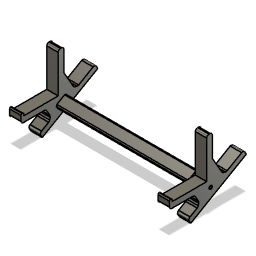
CHORDS Stand X2 (Autodesk Fusion 360 design; units mm, degrees)
Autodesk Fusion 360 part; units mm, degrees
sketch "Sketch1" plane through (0, 0, 0) normal (1, 0, 0) x (0, 0, -1)
  line L0 (0, 0) -> (-60, 0) construction
  line L1 (-60, 0) -> (-60, 138.5) construction
  line L2 (-60, 138.5) -> (0, 138.5) construction
  line L3 (0, 138.5) -> (0, 0) construction
  line L4 (0, 0) -> (-60, 0)
  line L5 (-60, 0) -> (-60.2, 0)
  line L6 (-60.2, 0) -> (-60.2, 5)
  line L7 (-60.2, 5) -> (-65.2, 5)
  line L8 (-65.2, 5) -> (-65.2, -10)
  line L9 (0, 0) -> (0, 70)
  line L10 (0, 70) -> (10, 70)
  line L11 (10, 70) -> (10, 30)
  line L12 (10, 30) -> (30, -4.641)
  line L13 (-65.2, -10) -> (-21.6, -10)
  line L14 (30, -4.641) -> (64.641, 15.359)
  line L15 (30, -4.641) -> (65.2811, -4.641) construction
  line L16 (30, -4.641) -> (-60.7782, -57.0519) construction
  line L17 (-21.6, -10) -> (-11.0205, -28.3242)
  line L18 (-11.0205, -28.3242) -> (-32.6711, -40.8242)
  line L19 (-32.6711, -40.8242) -> (-27.6711, -49.4845)
  line L20 (64.641, 15.359) -> (69.641, 6.6987)
  line L21 (69.641, 6.6987) -> (-27.6711, -49.4845)
  line L22 (0, 0) -> (14.5096, -25.1314) construction
  line L23 (14.5096, -25.1314) -> (9.5096, -16.4711) construction
  line L24 (9.5096, -16.4711) -> (18.1699, -11.4711)
  line L25 (18.1699, -11.4711) -> (13.1699, -2.8109)
  line L26 (13.1699, -2.8109) -> (4.5096, -7.8109)
  line L27 (-4.1506, -12.8109) -> (4.5096, -7.8109)
  line L28 (0.8494, -21.4711) -> (-4.1506, -12.8109)
  line L29 (9.5096, -16.4711) -> (0.8494, -21.4711)
  line L30 (-3.8774, -12.8841) -> (4.6096, -7.9841)
  line L31 (13.0967, -3.0841) -> (4.6096, -7.9841)
  line L32 (17.8967, -11.3979) -> (13.0967, -3.0841)
  line L33 (9.4096, -16.2979) -> (17.8967, -11.3979)
  line L34 (9.4096, -16.2979) -> (0.9226, -21.1979)
  line L35 (0.9226, -21.1979) -> (-3.8774, -12.8841)
  line L36 (4.5096, -7.8109) -> (9.5096, -16.4711) construction
  circle A0 centre (7.0096, -12.141) radius 2
  circle A1 centre (7.0096, -12.141) radius 1.85
  circle A2 centre (7.0096, -12.141) radius 2.5
  dimension "d1" = 60
  dimension "d2" = 138.5
  dimension "d3" = 0.2
  dimension "d4" = 5
  dimension "d5" = 5
  dimension "d6" = 15
  dimension "d7" = 70
  dimension "d8" = 10
  dimension "d9" = 40
  dimension "d10" = 150
  dimension "d11" = 40
  dimension "d12" = 43.6
  dimension "d13" = 30
  dimension "d14" = 40
  dimension "d15" = 25
  dimension "d16" = 10
  dimension "d17" = 10
  dimension "d18" = 10
  dimension "d19" = 10
  dimension "d20" = 10
  dimension "d21" = 0.2
  dimension "d22" = 4
  dimension "d23" = 3.7
  dimension "d26" = 5
  constraint horizontal L0
  constraint vertical L1
  constraint horizontal L2
  constraint vertical L3
  constraint coincident L0.start L3.end
  constraint perpendicular L1 L5
  constraint perpendicular L5 L6
  constraint perpendicular L6 L7
  constraint perpendicular L7 L8
  constraint coincident L3 L9.end
  constraint perpendicular L3 L10
  constraint perpendicular L10 L11
  constraint perpendicular L8 L13
  constraint horizontal L15
  constraint perpendicular L12 L16
  constraint coincident L16 L17.end
  constraint perpendicular L16 L17
  constraint coincident L16 L18.end
  constraint perpendicular L16 L19
  constraint perpendicular L14 L20
  constraint coincident L21 L22.end
  constraint perpendicular L21 L22
  constraint coincident L22 L23.end
  constraint perpendicular L23 L24
  constraint perpendicular L16 L25
  constraint coincident L22 L26.end
  constraint perpendicular L22 L26
  constraint symmetric L22 L23.end L24.start
  constraint symmetric L22 L24.end L28.start
  constraint symmetric L22 L25.end L27.start
  constraint symmetric L22 L26.end L27.end
  constraint midpoint L36 A0.centre
  constraint concentric A0 A1
  constraint concentric A1 A2
  measures "d1" distance of L0.start L0.end
  measures "d2" distance of L0.start L2.end
  measures "d3" distance of L0.end L5.end
  measures "d4" distance of L5.end L6.end
  measures "d5" distance of L6.end L7.end
  measures "d6" distance of L7.end L8.end
  measures "d7" distance of L0.start L9.end
  measures "d8" distance of L9.end L10.end
  measures "d9" distance of L10.end L11.end
  measures "d10" angle of L11 L12
  measures "d11" distance of L11.end L12.end
  measures "d12" distance of L8.end L13.end
  measures "d13" angle of L14 L15
  measures "d14" distance of L12.end L14.end
  measures "d15" distance of L17.end L18.end
  measures "d16" distance of L18.end L19.end
  measures "d17" distance of L14.end L20.end
  measures "d18" distance of L22.end L23.end
  measures "d19" distance of L23.end L24.end
  measures "d20" distance of L24.end L25.end
  measures "d22" diameter of A0
  measures "d23" diameter of A1
  measures "d26" diameter of A2
extrude "Extrude1" add sketch "Sketch1" along normal blind 20 contours L4 L5 L6 L7 L8 L9 L10 L11 L12 L13 L14 L17 L18 L19 L20 L21 makes body 1
extrude "Extrude2" add sketch "Sketch1" along normal blind 10 contours L24 L25 L26 L27 L28 L29 | L30 L31 L32 L33 L34 L35 | A0 | A2 bodies 1
extrude "Extrude3" cut sketch "Sketch1" along normal blind 3 contours A0 | A2 bodies 1
extrude "Extrude4" add sketch "Sketch1" along normal blind 240 from surface at 10 separate body contours L30 L31 L32 L33 L34 L35 | A2 makes body 2
extrude "Extrude5" add sketch "Sketch1" along normal blind 200 from surface at 30 contours A0 | A1 bodies 2
chamfer "Chamfer1" distance 2 angle 45 4 edges at (130, -3.0841, -13.0967) (130, -12.8841, 3.8774) (130, -21.1979, -0.9226) (130, -11.3979, -17.8967) on bodies 2
chamfer "Chamfer2" distance 2 angle 45 4 edges at (15, -2.8109, -13.1699) (15, -21.4711, -0.8494) (15, -12.8109, 4.1506) (15, -11.4711, -18.1699) on bodies 1
chamfer "Chamfer3" distance 5 angle 45 2 edges at (10, -28.3242, 11.0205) (10, -4.641, -30) on bodies 1
fillet "Fillet1" radius 4 11 edges at (10, -23.9941, 13.5205) (10, -30.8242, 15.3506) (10, -10, 21.6) (10, -10, 65.2) (10, 70, 0) (10, 70, -10) (10, 30, -10) (10, -0.3109, -27.5) (10, -2.141, -34.3301) (10, 15.359, -64.641) (10, -40.8242, 32.6711) on bodies 1
fillet "Fillet2" radius 2 2 edges at (10, 5, 65.2) (10, 5, 60.2) on bodies 1
chamfer "Chamfer4" distance 0.4 angle 45 2 edges at (0, -21.3929, -20.9849) (20, -21.3929, -20.9849) on bodies 1
chamfer "Chamfer5" distance 0.4 angle 45 1 edges at (0, -13.0451, -4.6788) on bodies 1
chamfer "Chamfer6" distance 1 angle 45 2 edges at (10, -12.8642, -5.145) (250, -11.4178, -5.145) on bodies 2
mirror "Mirror1" about plane through (0, 0, 0) normal (1, 0, 0) of bodies 1 makes body 3
move_body "Move1" bodies 3 to x (1, 0, 0) y (0, 1, 0) z (0, 0, 1) at (280, 0, 0)
equation "d10 = 90 deg + 60 deg"
equation "d12 = 5.6 mm + 38 mm"
